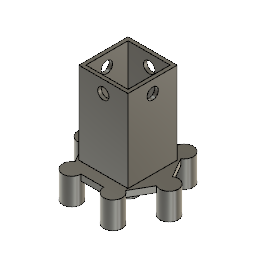
ExtrusionRack_Feet_standing_version (Autodesk Fusion 360 design; units mm, degrees)
Autodesk Fusion 360 part; units mm, degrees
note: some values were not read from the file. Set by a fixed rule: which sketch regions a step uses.
sketch "Sketch1" plane through (0, 0, 0) normal (0, 0, 1) x (1, 0, 0)
  circle A0 centre (0, 0) radius 5
  line L0 (10, 17.3205) -> (-10, 17.3205)
  line L1 (-10, 17.3205) -> (-20, 0)
  line L2 (-20, 0) -> (-10, -17.3205)
  line L3 (-10, -17.3205) -> (10, -17.3205)
  line L4 (10, -17.3205) -> (20, 0)
  line L5 (20, 0) -> (10, 17.3205)
  circle A1 centre (10, 17.3205) radius 4.5
  circle A2 centre (20, 0) radius 4.5
  circle A3 centre (10, -17.3205) radius 4.5
  circle A4 centre (-10, -17.3205) radius 4.5
  circle A5 centre (-20, 0) radius 4.5
  circle A6 centre (-10, 17.3205) radius 4.5
  dimension "d1" = 10
  dimension "d2" = 20
  dimension "d3" = 9
  dimension "d4" = 9
  dimension "d5" = 9
  dimension "d6" = 9
  dimension "d7" = 9
  dimension "d8" = 9
  constraint coincident A0.centre origin
  constraint horizontal L0
  constraint coincident L0.start L5.end
  constraint coincident L4.end L5.start
  constraint coincident L3.end L4.start
  constraint coincident L2.end L3.start
  constraint coincident L1.end L2.start
  constraint coincident L0.end L1.start
  measures "d1" diameter of A0
  measures "d2" distance of L0.start A0.centre
  measures "d3" diameter of A1
  measures "d4" diameter of A2
  measures "d5" diameter of A3
  measures "d6" diameter of A4
  measures "d7" diameter of A5
  measures "d8" diameter of A6
extrude "Extrude1" add sketch "Sketch1" against normal blind 10 contours A0 | L0 L1 A6 | L0 L1 A6 | L0 L5 A1 | L0 L5 A1 | L1 L2 A5 | L1 L2 A5 | L4 L5 A2 | L4 L5 A2 | L2 L3 A4 | L2 L3 A4 | L3 L4 A3 | L3 L4 A3 makes body 1 at (-5.5224, 17.7686, -3.3333) makes body 2 at (14.4776, -16.8725, -3.3333) makes body 3 at (14.4776, 17.7686, -3.3333) makes body 4 at (-15.5224, 0.4481, -3.3333) makes body 5 at (-5.5224, -16.8725, -3.3333) makes body 6 at (24.4944, -0.2243, -6.6667) makes body 7 at (4.9938, -0.2492, -6.6667)
extrude "Extrude2" add sketch "Sketch1" along normal blind 3 contours A0 | L0 L1 A6 | L0 L1 A6 | L0 L1 L2 L3 L4 L5 A1 A2 A3 A4 A5 A6 | L0 L5 A1 | L0 L5 A1 | L1 L2 A5 | L1 L2 A5 | L4 L5 A2 | L4 L5 A2 | L2 L3 A4 | L2 L3 A4 | L3 L4 A3 | L3 L4 A3 bodies 1 7 2 3 4 5 6
sketch "Sketch2" plane through (0, 0, 3) normal (0, 0, 1) x (1, 0, 0)
  line L0 (10.25, -10.25) -> (-10.25, -10.25)
  line L1 (-10.25, -10.25) -> (-10.25, 10.25)
  line L2 (-10.25, 10.25) -> (10.25, 10.25)
  line L3 (10.25, 10.25) -> (10.25, -10.25)
  line L4 (10.25, -10.25) -> (-10.25, 10.25) construction
  line L5 (-10.25, -10.25) -> (10.25, 10.25) construction
  line L6 (12, -12) -> (-12, -12)
  line L7 (-12, -12) -> (-12, 12)
  line L8 (-12, 12) -> (12, 12)
  line L9 (12, 12) -> (12, -12)
  line L10 (12, -12) -> (-12, 12) construction
  line L11 (-12, -12) -> (12, 12) construction
  arc A0 (-5.5, 17.3205) -> (-12.25, 13.4234) centre (-10, 17.3205) ccw
  line L12 (-12.25, 13.4234) -> (-17.75, 3.8971)
  arc A1 (-17.75, 3.8971) -> (-17.75, -3.8971) centre (-20, 0) ccw
  line L13 (-17.75, -3.8971) -> (-12.25, -13.4234)
  arc A2 (-12.25, -13.4234) -> (-5.5, -17.3205) centre (-10, -17.3205) ccw
  line L14 (-5.5, -17.3205) -> (5.5, -17.3205)
  arc A3 (5.5, -17.3205) -> (12.25, -13.4234) centre (10, -17.3205) ccw
  line L15 (12.25, -13.4234) -> (17.75, -3.8971)
  arc A4 (17.75, -3.8971) -> (17.75, 3.8971) centre (20, 0) ccw
  line L16 (17.75, 3.8971) -> (12.25, 13.4234)
  arc A5 (12.25, 13.4234) -> (5.5, 17.3205) centre (10, 17.3205) ccw
  line L17 (5.5, 17.3205) -> (-5.5, 17.3205)
  dimension "d13" = 20.5
  dimension "d14" = 20.5
  dimension "d15" = 24
  dimension "d16" = 24
  constraint perpendicular L0 L1
  constraint parallel L0 L2
  constraint parallel L1 L3
  constraint horizontal L0
  constraint coincident L4 origin
  constraint coincident L5 origin
  constraint perpendicular L6 L7
  constraint parallel L6 L8
  constraint parallel L7 L9
  constraint horizontal L6
  constraint coincident L10 origin
  constraint coincident L11 origin
  measures "d13" distance of L0.end L1.end
  measures "d14" distance of L1.end L2.end
  measures "d15" distance of L7.end L8.end
  measures "d16" distance of L6.end L7.end
extrude "Extrude3" add sketch "Sketch2" along normal blind 40 contours L6 L7 L8 L9 bodies 1
sketch "Sketch3" plane through (12, 0, 0) normal (1, 0, 0) x (0, 1, 0)
  line L0 (-12, 3) -> (12, 3)
  line L1 (12, 3) -> (12, 43)
  line L2 (12, 43) -> (-12, 43)
  line L3 (-12, 43) -> (-12, 3)
  circle A0 centre (0, 37) radius 2.75
  dimension "d19" = 5.5
  measures "d19" diameter of A0
extrude "Extrude4" cut sketch "Sketch3" against normal blind 31 contours A0 bodies 1
pattern_circular "C-Pattern1" count 4 over 360 about axis through (0, 0, 1.75) along (0, 0, 1) of "Extrude4"
